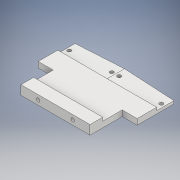
# Autodesk Inventor part: 앞뒷면PSD받침대_수정
Saved by Autodesk Inventor 2017 (Build 210142000, 142)
## iProperties
Part Number: 앞뒷면PSD받침대_수정
Material: ABS 플라스틱
Document SubType Name: Modeling
Designer: minom
Mass: 12.9687 g
Surface Area: 93.8696 cm^2
Volume: 12.2346 cm^3
Density: 1.06 g/cm^3
Appearance: 매끄러움 - 흰색
Author: minom
Autodesk Inventor part; units mm, degrees
ref_plane "YZ Plane" through (0, 0, 0) normal (1, 0, 0) x (0, 1, 0)
ref_plane "XZ Plane" through (0, 0, 0) normal (0, 1, 0) x (-1, 0, 0)
ref_plane "XY Plane" through (0, 0, 0) normal (0, 0, 1) x (1, 0, 0)
sketch "스케치1" plane through (0, 0, 0) normal (0, 0, 1) x (1, 0, 0)
  line L0 (0, 0) -> (60, 0)
  line L1 (60, 0) -> (60, 25)
  line L2 (60, 57) -> (0, 57)
  line L3 (0, 25) -> (0, 0)
  line L4 (-13, 57) -> (73, 57)
  line L5 (73, 57) -> (73, 25)
  line L6 (-13, 25) -> (-13, 57)
  line L7 (73, 25) -> (60, 25)
  line L8 (0, 25) -> (-13, 25)
  dimension "d0" = 60
  dimension "d1" = 57
  dimension "d3" = 86
  dimension "d4" = 32
  dimension "d5" = 13
  constraints: 18 end point, 5 parallel, 2 horizontal, 2 perpendicular
  measures "d0" distance of L2.end L2.start
  measures "d1" distance of L2.start L0.end
  measures "d3" distance of L5.end L6.start
  measures "d4" distance of L4.end L5.end
  measures "d5" distance between parallel lines of L3 L6
extrude "돌출1" add sketch "스케치1" along normal blind 8
sketch "스케치2" plane through (0, 0, 8) normal (0, 0, 1) x (1, 0, 0)
  line L0 (0, 0) -> (60, 0) projected
  line L1 (60, 0) -> (60, 25) projected
  line L2 (60, 25) -> (73, 25) projected
  line L3 (73, 25) -> (73, 57) projected
  line L4 (73, 57) -> (-13, 57) projected
  line L5 (-13, 57) -> (-13, 25) projected
  line L6 (-13, 25) -> (0, 25) projected
  line L7 (0, 25) -> (0, 0) projected
  line L8 (0, 25) -> (0, 0) projected
  line L9 (0, 8) -> (60, 8)
  line L10 (60, 8) -> (60, 0)
  line L11 (60, 0) -> (0, 0)
  line L12 (0, 0) -> (0, 8)
  dimension "d9" = 8
  dimension "d10" = 0
  constraints: 8 end point, 2 parallel, 2 point on line, 1 horizontal, 1 perpendicular
  measures "d9" distance of L9.end L10.end
  measures "d10" distance between parallel lines of L0 L11
extrude "돌출2" cut sketch "스케치2" against normal blind 3 contours L7 L6 L5 L4 L3 L2 L1 L9
sketch "스케치4" plane through (0, 0, 0) normal (0, -1, 0) x (1, 0, 0)
  line L0 (0, 0) -> (60, 0) projected
  line L1 (60, 0) -> (60, 8) projected
  line L2 (0, 8) -> (60, 8) projected
  line L3 (0, 0) -> (0, 8) projected
  circle A0 centre (45, 4) radius 1.5
  circle A1 centre (15, 4) radius 1.5
  dimension "d15" = 3
  dimension "d16" = 3
  dimension "d17" = 4
  dimension "d18" = 15
  dimension "d19" = 4
  dimension "d20" = 15
  constraints: 2 centre point
  measures "d15" diameter of A0
  measures "d16" diameter of A1
  measures "d17" distance from line of L0 A0.centre
  measures "d18" distance from line of L1 A0.centre
  measures "d19" distance from line of L2 A1.centre
  measures "d20" distance from line of L3 A1.centre
extrude "돌출4" cut sketch "스케치4" against normal blind 6 contours A0 | A1
sketch "스케치11" plane through (-13, 57, 5) normal (0, 1, 0) x (1, 0, 0)
  line L0 (0, 0) -> (86, 0) projected
  line L1 (86, 5) -> (86, 0) projected
  line L2 (86, 5) -> (0, 5) projected
  line L3 (0, 5) -> (0, 0) projected
  line L4 (0, 2.5) -> (43, 0)
  line L5 (0, 0) -> (86, 0) projected
  line L6 (73, 5) -> (86, 5) projected
  line L7 (43, 0) -> (43, 2.5)
  line L8 (86, 5) -> (0, 5) projected
  line L9 (86, 5) -> (43, 2.5)
  line L10 (0, 5) -> (43, 2.5)
  line L11 (43, 0) -> (86, 2.5)
  line L12 (86, 5) -> (86, 0) projected
  line L13 (86, 2.5) -> (86, 5)
  point P0 (13, 5)
  constraints: 12 end point, 3 midpoint, 1 collinear, 1 parallel, 1 perpendicular
extrude "돌출7" cut sketch "스케치11" against normal blind 15 contours L3 L4 L0 | L11 L1 L0 | L10 L2 L9
sketch "스케치13" plane through (-13, 57, 2.5) normal (-0.058, 0, 0.9983) x (0.9983, 0, 0.058)
  circle A0 centre (3, -8) radius 1.6
  circle A1 centre (40, -8) radius 1.6
  line L0 (0, -15) -> (0, 0) projected
  line L1 (0, 0) -> (43.0726, 0) projected
  line L2 (42.9275, -15) -> (-0.1451, -15) projected
  point P0 (12.833, -57)
  dimension "d53" = 3.2
  dimension "d54" = 3.2
  dimension "d55" = 37
  dimension "d56" = 3
  dimension "d57" = 8
  dimension "d58" = 7
  constraints: 2 centre point
  measures "d53" diameter of A0
  measures "d54" diameter of A1
  measures "d55" distance of A1.centre A0.centre
  measures "d56" distance from line of A0.centre L0
  measures "d57" distance from line of L1 A0.centre
  measures "d58" distance from line of L2 A1.centre
extrude "돌출8" cut sketch "스케치13" against normal blind 3
sketch "스케치15" plane through (0, 0, 0) normal (0, -1, 0) x (1, 0, 0)
  circle A0 centre (45, 4) radius 1.5 projected
  circle A1 centre (15, 4) radius 1.5 projected
  line L0 (0, 0) -> (60, 0) projected
  line L1 (60, 0) -> (60, 8) projected
  line L2 (0, 8) -> (60, 8) projected
  line L3 (0, 0) -> (0, 8) projected
extrude "돌출11" add sketch "스케치15" along normal blind 3
sketch "스케치16" plane through (30, 42, 5) normal (0.058, 0, 0.9983) x (0.9983, 0, -0.058)
  circle A0 centre (40.0726, 7) radius 1.6
  circle A1 centre (3.0737, 7.28) radius 1.6
  line L0 (0, 15) -> (43.0726, 15) projected
  line L1 (43.0726, 15) -> (43.0726, 0) projected
  point P0 (-29.6592, -42)
  dimension "d71" = 3.2
  dimension "d72" = 3.2
  dimension "d73" = 8
  dimension "d74" = 7.72
  dimension "d75" = 37
  dimension "d76" = 3
  constraints: 2 centre point
  measures "d71" diameter of A0
  measures "d72" diameter of A1
  measures "d73" distance from line of L0 A0.centre
  measures "d74" distance from line of L0 A1.centre
  measures "d75" distance of A0.centre A1.centre
  measures "d76" distance from line of A0.centre L1
extrude "돌출12" cut sketch "스케치16" against normal blind 10
